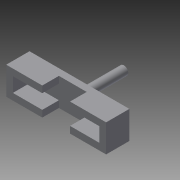
# Autodesk Inventor part: Side Clamp
Saved by Autodesk Inventor 2015 (Build 190159000, 159)
## iProperties
Created: 2016-11-04
Part Number: Side Clamp
Material: Generic
Document SubType Name: Modeling
Designer: william
Density: 1 g/cm^3
Appearance: Default
Author: william
Autodesk Inventor part; units mm, degrees
ref_plane "YZ Plane" through (0, 0, 0) normal (1, 0, 0) x (0, 1, 0)
ref_plane "XZ Plane" through (0, 0, 0) normal (0, 1, 0) x (-1, 0, 0)
ref_plane "XY Plane" through (0, 0, 0) normal (0, 0, 1) x (1, 0, 0)
sketch "Sketch1" plane through (0, 0, 0) normal (0, 1, 0) x (-1, 0, 0)
  line L0 (0, 0) -> (-90, 0)
  line L1 (-90, 0) -> (-90, 25)
  line L2 (-90, 25) -> (0, 25)
  line L3 (0, 25) -> (0, 0)
  dimension "d0" = 90
  dimension "d1" = 25
  constraints: 8 end point, 2 parallel, 1 horizontal, 1 perpendicular
  measures "d0" distance of L1.end L2.end
  measures "d1" distance of L0.end L1.end
extrude "Extrusion1" add sketch "Sketch1" along normal blind 21
sketch "Sketch2" plane through (0, 0, 0) normal (0, -1, 0) x (1, 0, 0)
  line L0 (0, 0) -> (90, 0) projected
  line L1 (90, 0) -> (90, 25) projected
  line L2 (90, 25) -> (0, 25) projected
  line L3 (0, 25) -> (0, 0) projected
  line L4 (6, 19) -> (84, 19)
  line L5 (84, 19) -> (84, 6)
  line L6 (84, 6) -> (6, 6)
  line L7 (6, 6) -> (6, 19)
  line L8 (90, 0) -> (0, 0) projected
  line L9 (32.5, 0) -> (32.5, 6)
  line L10 (32.5, 19) -> (32.5, 25)
  line L11 (57.5, 19) -> (57.5, 25)
  line L12 (57.5, 6) -> (57.5, 0)
  dimension "d4" = 6
  dimension "d10" = 25
  dimension "d11" = 25
  dimension "d12" = 78
  dimension "d13" = 26.5
  constraints: 16 end point, 10 point on line, 2 equal length, 1 perpendicular, 3 other
  measures "d4" distance between parallel lines of L2 L4
  measures "d10" distance between parallel lines of L12 L9
  measures "d11" distance between parallel lines of L11 L10
  measures "d12" distance of L4.start L4.end
  measures "d13" distance between parallel lines of L7 L10
extrude "Extrusion2" cut sketch "Sketch2" against normal blind 15 contours L9 L6 L12 L0 | L6 L7 L4 L5 | L2 L11 L4 L10
sketch "Sketch3" plane through (0, 21, 0) normal (0, 1, 0) x (1, 0, 0)
  circle A0 centre (45, -12.5) radius 4
  line L0 (0, 0) -> (0, -25) projected
  line L1 (0, -25) -> (90, -25) projected
  point P0 (0, -12.5)
  point P1 (45, -25)
  dimension "d7" = 8
  constraints: 2 midpoint, 1 centre point, 1 horizontal alignment, 1 vertical alignment
  measures "d7" diameter of A0
extrude "Extrusion3" add sketch "Sketch3" along normal blind 40
equation "\"d13\" = 0.5 * d12 - 0.5 * d11"
body "Solid1"
